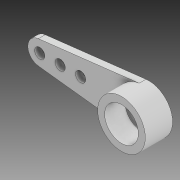
# Autodesk Inventor part: ServoHorn
Saved by Autodesk Inventor 2020 (Build 240168000, 168)
## iProperties
Created: 2021-05-16
Part Number: ServoHorn
Material: Generic
Document SubType Name: Modeling
Designer: DDeGo
Density: 1 g/cm^3
Appearance: Default
Author: DDeGo
Autodesk Inventor part; units mm, degrees
ref_plane "YZ Plane" through (0, 0, 0) normal (1, 0, 0) x (0, 1, 0)
ref_plane "XZ Plane" through (0, 0, 0) normal (0, 1, 0) x (-1, 0, 0)
ref_plane "XY Plane" through (0, 0, 0) normal (0, 0, 1) x (1, 0, 0)
sketch "Sketch1" plane through (0, 0, 0) normal (0, 0, 1) x (1, 0, 0)
  circle A0 centre (0, 0) radius 1.5
  circle A1 centre (-15, 0) radius 0.75
  line L0 (-15, 0) -> (0, 0) construction
  arc A2 (-0.4083, -3.4761) -> (-0.4083, 3.4761) centre (0, 0) ccw
  arc A3 (-15.2042, 1.738) -> (-15.2042, -1.738) centre (-15, 0) ccw
  circle A4 centre (-12, 0) radius 0.75
  circle A5 centre (-9, 0) radius 0.75
  line L1 (-15.2042, 1.738) -> (-0.4083, 3.4761)
  line L2 (-0.4083, -3.4761) -> (-15.2042, -1.738)
  dimension "d0" = 15
  dimension "d1" = 1.5
  dimension "d2" = 3
  dimension "d5" = 3
  dimension "d10" = 1
  dimension "d11" = 2
  constraints: 6 centre point, 6 end point, 4 point on circle, 4 tangent, 3 coincident, 2 horizontal, 4 other
  measures "d0" distance of L0.start L0.end
  measures "d1" diameter of A1
  measures "d2" diameter of A0
  measures "d5" distance of L0.start A4.centre
  measures "d10" radial gap between concentric circles of A3 A1
  measures "d11" radial gap between concentric circles of A2 A0
extrude "Extrusion1" add sketch "Sketch1" along normal blind 1
sketch "Sketch2" plane through (0, 0, 1) normal (0, 0, 1) x (1, 0, 0)
  arc A0 (-0.4083, -3.4761) -> (-0.4083, 3.4761) centre (0, 0) ccw projected
  circle A1 centre (0, 0) radius 3.5
  circle A2 centre (0, 0) radius 2.4727
  point P0 (-0.4083, -3.4761)
  constraints: 2 coincident, 1 centre point, 3 other
extrude "Extrusion2" add sketch "Sketch2" along normal blind 3
body "Solid1"
